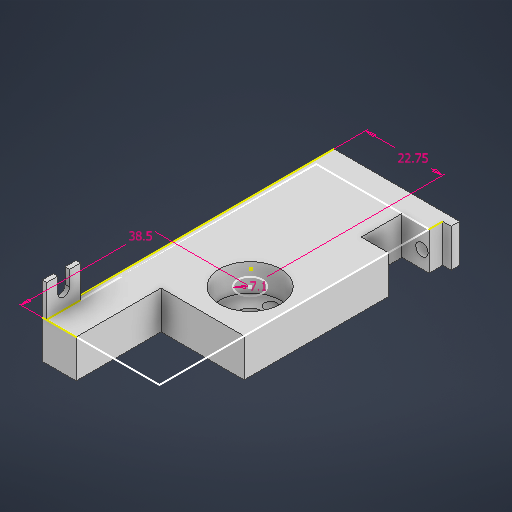
# Autodesk Inventor part: Knob Bracket
Saved by Autodesk Inventor 2026.2 (Build 302298000, 298)
## iProperties
Created: 2026-08-06
Part Number: Knob Bracket
Material: Generic
Document SubType Name: Modeling
Designer: Graeme
Density: 1 g/cm^3
Appearance: Default
Author: Graeme
## iProperties of the stored document Knob Bracket v4_3DPrint.ipt
Created: 2026-08-08
Part Number: Knob Bracket v4_3DPrint
Material: Generic
Document SubType Name: Modeling
Designer: Graeme
Density: 1 g/cm^3
Appearance: Default
Author: Graeme
Autodesk Inventor part; units mm, degrees
ref_plane "YZ Plane" through (0, 0, 0) normal (1, 0, 0) x (0, 1, 0)
ref_plane "XZ Plane" through (0, 0, 0) normal (0, 1, 0) x (-1, 0, 0)
ref_plane "XY Plane" through (0, 0, 0) normal (0, 0, 1) x (1, 0, 0)
sketch "Sketch1" plane through (0, 0, 0) normal (0, 1, 0) x (-1, 0, 0)
  line L0 (18.5, 43) -> (-18.5, 43)
  line L1 (-18.5, 43) -> (-18.5, -43)
  line L2 (-18.5, -43) -> (18.5, -43)
  line L3 (18.5, -43) -> (18.5, 43)
  line L4 (18.5, 43) -> (-18.5, -43) construction
  line L5 (-18.5, 43) -> (18.5, -43) construction
  point P0 (0, 0)
  dimension "d0" = 37
  dimension "d1" = 86
  constraints: 12 end point, 2 midpoint, 2 parallel, 1 horizontal, 1 perpendicular
  measures "d0" distance of L2.end L1.end
  measures "d1" distance of L1.end L0.end
extrude "Body" add sketch "Sketch1" along normal blind 11.2
sketch "Sketch2" plane through (18.5, 0, -43) normal (0, 0, -1) x (-1, 0, 0)
  circle A0 centre (32, 5) radius 1.85
  line L0 (37, 0) -> (37, 11.2) projected
  line L1 (0, 0) -> (37, 0) projected
  circle A1 centre (4.6, 5) radius 1.85
  line L2 (0, 0) -> (0, 11.2) projected
  point P0 (18.5, 0)
  dimension "d4" = 3.7
  dimension "d5" = 5
  dimension "d6" = 5
  dimension "d7" = 3.7
  dimension "d8" = 5
  dimension "d9" = 4.6
  constraints: 2 centre point
  measures "d4" diameter of A0
  measures "d5" distance from line of A0.centre L0
  measures "d6" distance from line of L1 A0.centre
  measures "d7" diameter of A1
  measures "d8" distance from line of L1 A1.centre
  measures "d9" distance from line of L2 A1.centre
extrude "Side Mounts" cut sketch "Sketch2" against normal blind 11.2
sketch "Sketch3" plane through (0, 11.2, 0) normal (0, 1, 0) x (1, 0, 0)
  line L0 (-18.5, -43) -> (18.5, -43) projected
  line L1 (18.5, 43) -> (16, 43)
  line L2 (16, 43) -> (16, -43)
  line L3 (16, -43) -> (18.5, -43)
  line L4 (18.5, -43) -> (18.5, 43)
  line L5 (16, 40.5) -> (18.5, 40.5)
  point P0 (0, 0)
  point P1 (17.25, 43)
  point P2 (17.25, 40.5)
  dimension "d12" = 2.5
  dimension "d13" = 2.5
  constraints: 10 end point, 3 point on line, 2 midpoint, 2 parallel, 2 perpendicular, 1 horizontal
  measures "d12" distance of L3.end L2.end
  measures "d13" distance of point (17.25, 43) point (17.25, 40.5)
extrude "mains cutout" cut sketch "Sketch3" against normal up to surface (11.2 mm away) contours L2 L5 L4 L0
sketch "Sketch4" plane through (0, 11.2, 0) normal (0, 1, 0) x (1, 0, 0)
  line L0 (16, 40.5) -> (16, -43) projected
  line L1 (-18.5, -43) -> (-8.5, -43)
  line L2 (-8.5, -43) -> (-8.5, -18)
  line L3 (-8.5, -18) -> (16, -18)
  line L4 (16, -43) -> (-8.5, -43)
  point P0 (0, 0)
  dimension "d19" = 25
  constraints: 8 end point, 3 perpendicular, 1 horizontal, 1 point on line
  measures "d19" distance of L2.end L1.end
extrude "screen cut out" cut sketch "Sketch4" against normal up to surface (11.2 mm away)
sketch "Sketch5" plane through (0, 11.2, 0) normal (0, 1, 0) x (1, 0, 0)
  line L0 (-18.5524, -42.9481) -> (-17.2524, -42.9481)
  line L1 (-17.2524, -42.9481) -> (-17.2524, -32.9481)
  line L2 (-17.2524, -32.9481) -> (-18.5524, -32.9481)
  line L3 (-18.5524, -32.9481) -> (-18.5524, -42.9481)
  point P0 (0, 0)
  dimension "d22" = 1.3
  dimension "d23" = 10
  constraints: 8 end point, 2 parallel, 1 horizontal, 1 perpendicular
  measures "d22" distance of L2.end L1.end
  measures "d23" distance of L1.end L0.end
extrude "top mount bracket" add sketch "Sketch5" along normal blind 9.5
sketch "Sketch6" plane through (-18.5524, 11.2, 32.9481) normal (-1, 0, 0) x (0, 0, 1)
  circle A0 centre (5, 5) radius 1.75
  line L0 (0, 9.5) -> (10, 9.5) projected
  line L1 (0, 0) -> (0, 9.5) projected
  line L2 (3.25, 5) -> (3.25, 9.5)
  line L3 (6.75, 9.5) -> (6.75, 5)
  point P0 (-32.9481, -11.2)
  dimension "d26" = 3.5
  dimension "d27" = 4.5
  dimension "d28" = 5
  constraints: 4 end point, 2 point on circle, 2 point on line, 1 centre point, 1 parallel, 1 perpendicular, 1 tangent
  measures "d26" diameter of A0
  measures "d27" distance from line of L0 A0.centre
  measures "d28" distance from line of L1 A0.centre
extrude "top mount hole" cut sketch "Sketch6" against normal up to surface (1.3 mm away)
sketch "Sketch7" plane through (0, 11.2, 0) normal (0, 1, 0) x (1, 0, 0)
  circle A0 centre (4.25, -4.5) radius 3.55
  line L0 (-18.5, 43) -> (-18.5, -32.9481) projected
  line L1 (-18.5, -43) -> (-8.5, -43) projected
  point P0 (0, 0)
  dimension "d32" = 7.1
  dimension "d33" = 22.75
  dimension "d34" = 38.5
  constraints: 1 centre point
  measures "d32" diameter of A0
  measures "d33" distance from line of L0 A0.centre
  measures "d34" distance from line of A0.centre L1
extrude "Pot hole" cut sketch "Sketch7" against normal up to surface (11.2 mm away)
sketch "Sketch8" plane through (0, 11.2, 0) normal (0, 1, 0) x (1, 0, 0)
  circle A0 centre (4.25, -4.5) radius 9
  point P0 (0, 0)
  dimension "d37" = 18
  constraints: 1 centre point, 1 coincident
  measures "d37" diameter of A0
extrude "Extrusion8" cut sketch "Sketch8" against normal blind 8
sketch "Sketch9" plane through (0, 11.2, 0) normal (0, 1, 0) x (1, 0, 0)
  line L0 (16, -18) -> (16, 40.5) projected
  line L1 (16, 40.5) -> (16, 28.5)
  line L2 (16, 40.5) -> (16, 36.5)
  line L3 (16, 36.5) -> (8, 36.5)
  line L4 (8, 36.5) -> (8, 24.5)
  line L5 (8, 24.5) -> (16, 24.5)
  line L6 (16, 24.5) -> (16, 36.5)
  point P0 (0, 0)
  dimension "d42" = 4
  dimension "d43" = 8
  dimension "d44" = 12
  constraints: 12 end point, 2 parallel, 2 point on line, 1 horizontal, 1 perpendicular
  measures "d42" distance of L0.end L2.end
  measures "d43" distance of L5.end L4.end
  measures "d44" distance of L4.end L3.end
extrude "Extrusion9" cut sketch "Sketch9" against normal up to surface (11.2 mm away)
sketch "Sketch10" plane through (0, 11.2, 0) normal (0, 1, 0) x (1, 0, 0)
  line L0 (16, 36.5) -> (16, 40.5) projected
  line L1 (-17.2524, -32.9481) -> (-17.2524, -42.9481) projected
  line L2 (16, 36.5) -> (-17.2524, 36.5)
  line L3 (-17.2524, 36.5) -> (-17.2524, -42.9481)
  line L4 (-17.2524, -42.9481) -> (16, -42.9481)
  line L5 (16, -42.9481) -> (16, 36.5)
  point P0 (0, 0)
  constraints: 8 end point, 2 parallel, 1 horizontal, 1 perpendicular
sketch "encoder locator" plane through (0, 0, 0) normal (0, -1, 0) x (1, 0, 0)
  line L0 (4.25, 4.5) -> (4.25, -1.5)
  circle A0 centre (4.25, -1.5) radius 1.75
  point P0 (0, 0)
  dimension "d49" = 6
  dimension "d50" = 3.5
  constraints: 2 coincident, 2 end point, 1 centre point, 1 vertical
  measures "d49" distance of L0.start L0.end
  measures "d50" diameter of A0
extrude "Extrusion11" cut sketch "encoder locator" against normal up to surface (3.2 mm away)
equation "\"d8\" = d6"
body "Solid1"
